Autodesk Fusion 360 part; units mm, degrees
(part 2 of 2)
sketch "Sketch5" plane through (-68.5, 0, 0) normal (-1, 0, 0) x (0, -1, 0) in component "Side"
  line L0 (-67.55, 105) -> (-67.55, 160)
  line L1 (-67.55, 160) -> (-77.55, 160)
  line L2 (-77.55, 160) -> (-77.55, 10)
  line L3 (-77.55, 10) -> (55.8, 10)
  line L4 (55.8, 10) -> (55.8, 20)
  line L5 (55.8, 20) -> (35.4, 20)
  arc A0 (20.4, 35) -> (35.4, 20) centre (35.4, 35) ccw
  line L6 (20.4, 35) -> (20.4, 88)
  arc A1 (20.4, 88) -> (18.4, 90) centre (18.4, 88) ccw
  line L7 (18.4, 90) -> (17.9998, 90)
  arc A2 (14.9998, 93) -> (17.9998, 90) centre (17.9998, 93) ccw
  line L8 (14.9998, 93) -> (14.9998, 112)
  arc A3 (14.9998, 112) -> (11.9998, 115) centre (11.9998, 112) ccw
  line L9 (11.9998, 115) -> (4.9998, 115)
  line L10 (4.9998, 115) -> (4.9998, 100)
  arc A4 (-5.0002, 100) -> (4.9998, 100) centre (-0.0002, 100) ccw
  line L11 (-5.0002, 100) -> (-5.0002, 115)
  line L12 (-5.0002, 115) -> (-12.0002, 115)
  arc A5 (-12.0002, 115) -> (-15.0002, 112) centre (-12.0002, 112) ccw
  line L13 (-15.0002, 112) -> (-15.0002, 95)
  arc A6 (-20.0002, 90) -> (-15.0002, 95) centre (-20.0002, 95) ccw
  line L14 (-20.0002, 90) -> (-52.55, 90)
  arc A7 (-67.55, 105) -> (-52.55, 90) centre (-52.55, 105) ccw
  line L15 (-0.0002, 95) -> (-0.0002, 10) construction
  line L16 (-25.4002, 90) -> (-25.4002, 10) construction
  line L17 (-50.8002, 90) -> (-50.8002, 10) construction
  line L18 (20.4, 30.4257) -> (-77.55, 30.4257) construction
  line L19 (20.4, 55.8257) -> (-77.55, 55.8257) construction
  line L20 (20.4, 81.2257) -> (-77.55, 81.2257) construction
  line L21 (-0.0002, 81.2257) -> (-50.8002, 30.4257) construction
  line L22 (-50.8002, 81.2257) -> (-0.0002, 30.4257) construction
  line L23 (-50.8002, 55.8257) -> (-25.4002, 81.2257) construction
  line L24 (-25.4002, 30.4257) -> (-0.0002, 55.8257) construction
  line L25 (-50.8002, 55.8257) -> (-25.4002, 30.4257) construction
  line L26 (-25.4002, 81.2257) -> (-0.0002, 55.8257) construction
  line L27 (-50.8002, 68.5257) -> (-0.0002, 68.5257) construction
  line L28 (-38.1002, 81.2257) -> (-38.1002, 30.4257) construction
  line L29 (-12.7002, 30.4257) -> (-12.7002, 81.2257) construction
  line L30 (-50.8002, 43.1257) -> (-0.0002, 43.1257) construction
  circle A8 centre (-50.8002, 81.2257) radius 3.1375
  circle A9 centre (-25.4002, 81.2257) radius 3.1375
  circle A10 centre (-0.0002, 81.2257) radius 3.1375
  circle A11 centre (-50.8002, 68.5257) radius 3.1375
  circle A12 centre (-25.4002, 68.5257) radius 3.1375
  circle A13 centre (-0.0002, 68.5257) radius 3.1375
  circle A14 centre (-50.8002, 55.8257) radius 3.1375
  circle A15 centre (-25.4002, 55.8257) radius 3.1375
  circle A16 centre (-0.0002, 55.8257) radius 3.1375
  circle A17 centre (-50.8002, 43.1257) radius 3.1375
  circle A18 centre (-38.1002, 81.2257) radius 3.1375
  circle A19 centre (-12.7002, 81.2257) radius 3.1375
  circle A20 centre (-38.1002, 68.5257) radius 3.1375
  circle A21 centre (-12.7002, 68.5257) radius 3.1375
  circle A22 centre (-38.1002, 55.8257) radius 3.1375
  circle A23 centre (-12.7002, 55.8257) radius 3.1375
  circle A24 centre (-38.1002, 43.1257) radius 3.1375
  circle A25 centre (-25.4002, 43.1257) radius 3.1375
  circle A26 centre (-12.7002, 43.1257) radius 3.1375
  circle A27 centre (-0.0002, 43.1257) radius 3.1375
  circle A28 centre (-0.0002, 30.4257) radius 3.1375
  circle A29 centre (-12.7002, 30.4257) radius 3.1375
  circle A30 centre (-25.4002, 30.4257) radius 3.1375
  circle A31 centre (-38.1002, 30.4257) radius 3.1375
  circle A32 centre (-50.8002, 30.4257) radius 3.1375
  line L31 (-77.55, 160) -> (-46.5335, 160)
  line L32 (-46.5335, 160) -> (-46.5335, 35)
  line L33 (-46.5335, 35) -> (-77.55, 35)
  line L34 (-77.55, 35) -> (-77.55, 160)
  dimension "d151" = 25.4
  dimension "d152" = 25.4
  dimension "d155" = 25.4
  dimension "d156" = 25.4
  dimension "d157" = 6.275
  dimension "d159" = 6.275
  dimension "d161" = 6.275
  dimension "d162" = 6.275
  dimension "d164" = 6.275
  dimension "d166" = 6.275
  dimension "d167" = 6.275
  dimension "d169" = 6.275
  dimension "d171" = 6.275
  dimension "d172" = 6.275
  dimension "d173" = 12.7
  dimension "d174" = 12.7
  dimension "d175" = 12.7
  dimension "d176" = 12.7
  dimension "d177" = 6.275
  dimension "d178" = 6.275
  dimension "d179" = 6.275
  dimension "d180" = 6.275
  dimension "d181" = 6.275
  dimension "d182" = 6.275
  dimension "d183" = 6.275
  dimension "d184" = 6.275
  dimension "d185" = 6.275
  dimension "d186" = 6.275
  dimension "d187" = 6.275
  dimension "d188" = 6.275
  dimension "d189" = 6.275
  dimension "d190" = 6.275
  dimension "d191" = 6.275
  dimension "d361" = 125
  constraint midpoint A4 L15.start
  constraint coincident L3 L15.end
  constraint perpendicular L3 L15
  constraint coincident L14 L16.start
  constraint coincident L3 L16.end
  constraint perpendicular L3 L16
  constraint coincident L14 L17.start
  constraint coincident L3 L17.end
  constraint perpendicular L3 L17
  constraint coincident L6 L18.start
  constraint coincident L2 L18.end
  constraint perpendicular L2 L18
  constraint coincident L6 L19.start
  constraint coincident L2 L19.end
  constraint perpendicular L2 L19
  constraint coincident L6 L20.start
  constraint coincident L2 L20.end
  constraint perpendicular L2 L20
  constraint coincident L15 L21.start
  constraint coincident L20 L21.start
  constraint coincident L18 L21.end
  constraint coincident L17 L21.end
  constraint coincident L17 L22.start
  constraint coincident L20 L22.start
  constraint coincident L18 L22.end
  constraint coincident L15 L22.end
  constraint coincident L19 L23.start
  constraint coincident L17 L23.start
  constraint coincident L20 L23.end
  constraint coincident L16 L23.end
  constraint coincident L18 L24.start
  constraint coincident L16 L24.start
  constraint coincident L19 L24.end
  constraint coincident L15 L24.end
  constraint coincident L17 L27.start
  constraint coincident L15 L27.end
  constraint perpendicular L15 L27
  constraint coincident L20 L28.start
  constraint coincident L18 L28.end
  constraint perpendicular L18 L28
  constraint coincident L18 L29.start
  constraint coincident L20 L29.end
  constraint perpendicular L20 L29
  constraint coincident L17 L30.start
  constraint coincident L15 L30.end
  constraint perpendicular L15 L30
  constraint coincident L22.start A8.centre
  constraint coincident L23.end L26.start
  constraint coincident L21.start A10.centre
  constraint coincident L27.start A11.centre
  constraint midpoint L27 A12.centre
  constraint coincident L27.end A13.centre
  constraint coincident L23.start L25.start
  constraint midpoint L21 A15.centre
  constraint coincident L24.end L26.end
  constraint coincident L30.start A17.centre
  constraint coincident L28.start A18.centre
  constraint coincident L29.end A19.centre
  constraint midpoint L23 A20.centre
  constraint midpoint L26 A21.centre
  constraint midpoint L28 A22.centre
  constraint midpoint L29 A23.centre
  constraint midpoint L25 A24.centre
  constraint midpoint L30 A25.centre
  constraint coincident L30 A26.centre
  constraint coincident L29 A26.centre
  constraint coincident L30.end A27.centre
  constraint coincident L22.end A28.centre
  constraint coincident L29.start A29.centre
  constraint coincident L24.start L25.end
  constraint coincident L28.end A31.centre
  constraint coincident L21.end A32.centre
  constraint horizontal L31
  constraint vertical L32
  constraint horizontal L33
  constraint vertical L34
  constraint coincident L1.end L2.start
  measures "d151" distance of L15 L16
  measures "d152" distance of L16 L17
  measures "d155" distance of L19 L20
  measures "d156" distance of L18 L19
  measures "d157" diameter of A8
  measures "d159" diameter of A9
  measures "d161" diameter of A10
  measures "d162" diameter of A11
  measures "d164" diameter of A12
  measures "d166" diameter of A13
  measures "d167" diameter of A14
  measures "d169" diameter of A15
  measures "d171" diameter of A16
  measures "d172" diameter of A17
  measures "d173" distance of L17 L28
  measures "d174" distance of L16 L29
  measures "d175" distance of L20 L27
  measures "d176" distance of L19 L30
  measures "d177" diameter of A18
  measures "d178" diameter of A19
  measures "d179" diameter of A20
  measures "d180" diameter of A21
  measures "d181" diameter of A22
  measures "d182" diameter of A23
  measures "d183" diameter of A24
  measures "d184" diameter of A25
  measures "d185" diameter of A26
  measures "d186" diameter of A27
  measures "d187" diameter of A28
  measures "d188" diameter of A29
  measures "d189" diameter of A30
  measures "d190" diameter of A31
  measures "d191" diameter of A32
  measures "d361" distance of L1.end L33.end
extrude "Extrude5" cut sketch "Sketch5" against normal up to surface (10 mm away) contours A8 | A9 | A10 | A11 | A12 | A13 | A14 | A15 | A16 | A17 | A18 | A19 | A20 | A21 | A22 | A23 | A24 | A25 | A26 | A27 | A28 | A29 | A30 | A31 | A32 bodies 3 in component "Side"
sketch "Sketch6" plane through (0, -14.9998, 0) normal (0, -1, 0) x (1, 0, 0) in component "Side"
  line L0 (-58.5, 93) -> (-58.5, 112)
  line L1 (-58.5, 112) -> (-68.5, 112)
  line L2 (-68.5, 112) -> (-68.5, 93)
  line L3 (-68.5, 93) -> (-58.5, 93)
  line L4 (-58.5, 112) -> (-68.5, 93) construction
  line L5 (-68.5, 112) -> (-58.5, 93) construction
  circle A0 centre (-63.5, 102.5) radius 3.1375
  dimension "d194" = 6.275
  constraint coincident L0.end L1.start
  constraint coincident L2.end L3.start
  constraint coincident L1.end L2.start
  constraint coincident L0.start L3.end
  constraint midpoint L5 A0.centre
  measures "d194" diameter of A0
extrude "Extrude6" cut sketch "Sketch6" against normal up to surface (3 mm away) contours A0 bodies 3 in component "Side"
sketch "Sketch7" plane through (0, 77.55, 0) normal (0, 1, 0) x (-1, 0, 0) in component "Side"
  line L0 (58.5, 10) -> (68.5, 10)
  line L1 (68.5, 10) -> (68.5, 160)
  line L2 (68.5, 160) -> (58.5, 160)
  line L3 (58.5, 160) -> (58.5, 10)
  line L4 (68.5, 160) -> (58.5, 10) construction
  line L5 (58.5, 160) -> (68.5, 10) construction
  line L6 (58.5, 85) -> (68.5, 85) construction
  line L7 (58.5, 85) -> (68.5, 160) construction
  line L8 (58.5, 160) -> (68.5, 85) construction
  line L9 (68.5, 85) -> (58.5, 10) construction
  line L10 (58.5, 85) -> (68.5, 10) construction
  circle A0 centre (63.5, 47.5) radius 3.1375
  circle A1 centre (63.5, 85) radius 3.1375
  circle A2 centre (63.5, 122.5) radius 3.1375
  dimension "d197" = 6.275
  dimension "d198" = 6.275
  dimension "d199" = 6.275
  constraint coincident L1.end L2.start
  constraint coincident L0.start L3.end
  constraint coincident L2.end L3.start
  constraint coincident L0.end L1.start
  constraint midpoint L3 L6.start
  constraint midpoint L1 L6.end
  constraint midpoint L9 A0.centre
  constraint midpoint L4 A1.centre
  constraint midpoint L8 A2.centre
  measures "d197" diameter of A0
  measures "d198" diameter of A1
  measures "d199" diameter of A2
extrude "Extrude7" cut sketch "Sketch7" against normal blind 22.5 contours A0 | A1 | A2 bodies 3 in component "Side"
sketch "Sketch3 (2)" plane through (0, 77.55, 0) normal (0, -1, 0) x (1, 0, 0) in component "Back"
  line L0 (-68.5, 10) -> (68.5, 10)
  line L1 (68.5, 10) -> (68.5, 160)
  line L2 (68.5, 160) -> (-68.5, 160)
  line L3 (-68.5, 160) -> (-68.5, 10)
  line L4 (-58.5, 160) -> (-58.5, 10) construction
  line L5 (58.5, 160) -> (58.5, 10) construction
  line L6 (-58.5, 160) -> (-68.5, 10) construction
  line L7 (-68.5, 160) -> (-58.5, 10) construction
  line L8 (-68.5, 85) -> (-58.5, 160) construction
  line L9 (-68.5, 160) -> (-58.5, 85) construction
  line L10 (-58.5, 85) -> (-68.5, 10) construction
  line L11 (-68.5, 85) -> (-58.5, 10) construction
  circle A0 centre (-63.5, 47.5) radius 3.35
  line L12 (68.5, 160) -> (58.5, 10) construction
  line L13 (58.5, 160) -> (68.5, 10) construction
  line L14 (58.5, 85) -> (68.5, 160) construction
  line L15 (58.5, 160) -> (68.5, 85) construction
  line L16 (68.5, 85) -> (58.5, 10) construction
  line L17 (58.5, 85) -> (68.5, 10) construction
  circle A1 centre (63.5, 47.5) radius 3.35
  line L18 (0, 160) -> (0, 10) construction
  line L19 (25.4, 160) -> (25.4, 10) construction
  line L20 (50.8, 160) -> (50.8, 10) construction
  line L21 (-25.4, 160) -> (-25.4, 10) construction
  line L22 (-50.8, 160) -> (-50.8, 10) construction
  line L23 (-68.5, 147.9) -> (68.5, 147.9) construction
  line L24 (-63.5, 122.5) -> (63.5, 122.5) construction
  line L25 (-68.5, 97.1) -> (68.5, 97.1) construction
  line L26 (-68.5, 46.3) -> (68.5, 46.3) construction
  line L27 (-68.5, 20.9) -> (68.5, 20.9) construction
  line L28 (-68.5, 71.7) -> (68.5, 71.7) construction
  line L29 (-50.8, 147.9) -> (50.8, 46.3) construction
  line L30 (-50.8, 122.5) -> (50.8, 20.9) construction
  line L31 (50.8, 147.9) -> (-50.8, 46.3) construction
  line L32 (50.8, 122.5) -> (-50.8, 20.9) construction
  line L33 (25.4, 147.9) -> (-50.8, 71.7) construction
  line L34 (0, 147.9) -> (-50.8, 97.1) construction
  line L35 (-25.4, 147.9) -> (-50.8, 122.5) construction
  line L36 (-25.4, 147.9) -> (50.8, 71.7) construction
  line L37 (0, 147.9) -> (50.8, 97.1) construction
  line L38 (25.4, 147.9) -> (50.8, 122.5) construction
  line L39 (-50.8, 97.1) -> (25.4, 20.9) construction
  line L40 (-50.8, 71.7) -> (0, 20.9) construction
  line L41 (-50.8, 46.3) -> (-25.4, 20.9) construction
  line L42 (-25.4, 20.9) -> (50.8, 97.1) construction
  line L43 (0, 20.9) -> (50.8, 71.7) construction
  line L44 (25.4, 20.9) -> (50.8, 46.3) construction
  circle A2 centre (-50.8, 46.3) radius 3.1375
  circle A3 centre (-25.4, 46.3) radius 3.1375
  circle A4 centre (0, 46.3) radius 3.1375
  circle A5 centre (25.4, 46.3) radius 3.1375
  circle A6 centre (50.8, 46.3) radius 3.1375
  circle A7 centre (-50.8, 20.9) radius 3.1375
  circle A8 centre (-25.4, 20.9) radius 3.1375
  circle A9 centre (0, 20.9) radius 3.1375
  circle A10 centre (25.4, 20.9) radius 3.1375
  circle A11 centre (50.8, 20.9) radius 3.1375
  circle A12 centre (-38.1, 33.6) radius 3.1375
  circle A13 centre (-12.7, 33.6) radius 3.1375
  circle A14 centre (12.7, 33.6) radius 3.1375
  circle A15 centre (38.1, 33.6) radius 3.1375
  circle A16 centre (63.5, 47.5) radius 5
  circle A17 centre (-63.5, 47.5) radius 5
  dimension "d202" = 10
  dimension "d203" = 10
  dimension "d206" = 6.7
  dimension "d209" = 6.7
  dimension "d210" = 25.4
  dimension "d211" = 25.4
  dimension "d212" = 25.4
  dimension "d213" = 25.4
  dimension "d214" = 25.4
  dimension "d215" = 25.4
  dimension "d216" = 25.4
  dimension "d217" = 25.4
  dimension "d218" = 25.4
  dimension "d239" = 6.275
  dimension "d240" = 6.275
  dimension "d241" = 6.275
  dimension "d242" = 6.275
  dimension "d243" = 6.275
  dimension "d244" = 6.275
  dimension "d245" = 6.275
  dimension "d246" = 6.275
  dimension "d247" = 6.275
  dimension "d248" = 6.275
  dimension "d265" = 6.275
  dimension "d266" = 6.275
  dimension "d267" = 6.275
  dimension "d268" = 6.275
  dimension "d351" = 10
  dimension "d354" = 10
  constraint coincident L2 L4.start
  constraint coincident L0 L4.end
  constraint perpendicular L0 L4
  constraint coincident L2 L5.start
  constraint coincident L0 L5.end
  constraint perpendicular L0 L5
  constraint coincident L0.start L3.end
  constraint coincident L2.end L3.start
  constraint midpoint L3 L8.start
  constraint midpoint L1 L15.end
  constraint midpoint L4 L9.end
  constraint midpoint L11 A0.centre
  constraint coincident L1.end L2.start
  constraint coincident L0.end L1.start
  constraint midpoint L5 L14.start
  constraint midpoint L17 A1.centre
  constraint midpoint L2 L18.start
  constraint midpoint L0 L18.end
  constraint coincident L2 L19.start
  constraint coincident L0 L19.end
  constraint perpendicular L0 L19
  constraint coincident L2 L20.start
  constraint coincident L0 L20.end
  constraint perpendicular L0 L20
  constraint coincident L2 L21.start
  constraint coincident L0 L21.end
  constraint perpendicular L0 L21
  constraint coincident L2 L22.start
  constraint coincident L0 L22.end
  constraint perpendicular L0 L22
  constraint coincident L3 L23.start
  constraint coincident L1 L23.end
  constraint perpendicular L1 L23
  constraint coincident L3 L25.start
  constraint coincident L1 L25.end
  constraint perpendicular L1 L25
  constraint coincident L3 L26.start
  constraint coincident L1 L26.end
  constraint perpendicular L1 L26
  constraint coincident L3 L27.start
  constraint coincident L1 L27.end
  constraint perpendicular L1 L27
  constraint coincident L3 L28.start
  constraint coincident L1 L28.end
  constraint perpendicular L1 L28
  constraint coincident L23 L29.start
  constraint coincident L22 L29.start
  constraint coincident L26 L29.end
  constraint coincident L20 L29.end
  constraint coincident L22 L30.start
  constraint coincident L24 L30.start
  constraint coincident L27 L30.end
  constraint coincident L20 L30.end
  constraint coincident L23 L31.start
  constraint coincident L20 L31.start
  constraint coincident L26 L31.end
  constraint coincident L22 L31.end
  constraint coincident L20 L32.start
  constraint coincident L24 L32.start
  constraint coincident L22 L32.end
  constraint coincident L27 L32.end
  constraint coincident L19 L33.start
  constraint coincident L23 L33.start
  constraint coincident L28 L33.end
  constraint coincident L22 L33.end
  constraint midpoint L23 L34.start
  constraint coincident L25 L34.end
  constraint coincident L22 L34.end
  constraint coincident L23 L35.start
  constraint coincident L21 L35.start
  constraint coincident L28 L36.end
  constraint coincident L20 L36.end
  constraint coincident L25 L37.end
  constraint coincident L20 L37.end
  constraint coincident L27 L39.end
  constraint coincident L19 L39.end
  constraint midpoint L27 L40.end
  constraint coincident L21 L41.end
  constraint coincident L27 L41.end
  constraint coincident L31.end L41.start
  constraint midpoint L40 A3.centre
  constraint midpoint L26 A4.centre
  constraint midpoint L43 A5.centre
  constraint coincident L29.end L44.end
  constraint coincident L32.end A7.centre
  constraint coincident L41.end L42.start
  constraint coincident L40.end L43.start
  constraint coincident L39.end L44.start
  constraint coincident L30.end A11.centre
  constraint midpoint L41 A12.centre
  constraint coincident L42 A13.centre
  constraint coincident L40 A13.centre
  constraint coincident L43 A14.centre
  constraint coincident L39 A14.centre
  constraint midpoint L44 A15.centre
  constraint concentric A1 A16
  constraint concentric A0 A17
  measures "d202" distance of L3 L4
  measures "d203" distance of L1 L5
  measures "d206" diameter of A0
  measures "d209" diameter of A1
  measures "d210" distance of L18 L19
  measures "d211" distance of L19 L20
  measures "d212" distance of L18 L21
  measures "d213" distance of L21 L22
  measures "d214" distance of L23 L24
  measures "d215" distance of L24 L25
  measures "d216" distance of L25 L28
  measures "d217" distance of L26 L28
  measures "d218" distance of L26 L27
  measures "d239" diameter of A2
  measures "d240" diameter of A3
  measures "d241" diameter of A4
  measures "d242" diameter of A5
  measures "d243" diameter of A6
  measures "d244" diameter of A7
  measures "d245" diameter of A8
  measures "d246" diameter of A9
  measures "d247" diameter of A10
  measures "d248" diameter of A11
  measures "d265" diameter of A12
  measures "d266" diameter of A13
  measures "d267" diameter of A14
  measures "d268" diameter of A15
  measures "d351" diameter of A16
  measures "d354" diameter of A17
extrude "Extrude3'" cut sketch "Sketch3 (2)" against normal up to surface (10 mm away) contours A0 | A1 | A2 | A3 | A4 | A5 | A6 | A7 | A8 | A9 | A10 | A11 | A12 | A13 | A14 | A15 bodies 2 in component "Back"
sketch "Sketch1 (4)" plane through (0, 0, 10) normal (0, 0, 1) x (-1, 0, 0) in component "Plate"
  circle A0 centre (-12.7, 25.4) radius 3.1375
  circle A1 centre (12.7, 25.4) radius 3.1375
  line L0 (76.55, -65) -> (75.85, -65)
  arc A2 (72.85, -62) -> (75.85, -65) centre (75.85, -62) ccw
  line L1 (72.85, -62) -> (72.85, 62)
  arc A3 (75.85, 65) -> (72.85, 62) centre (75.85, 62) ccw
  line L2 (75.85, 65) -> (76.55, 65)
  arc A4 (79.55, 62) -> (76.55, 65) centre (76.55, 62) ccw
  line L3 (79.55, 62) -> (79.55, -62)
  arc A5 (76.55, -65) -> (79.55, -62) centre (76.55, -62) ccw
  arc A6 (-76.55, 65) -> (-79.55, 62) centre (-76.55, 62) ccw
  line L4 (-76.55, 65) -> (-75.85, 65)
  arc A7 (-72.85, 62) -> (-75.85, 65) centre (-75.85, 62) ccw
  line L5 (-72.85, 62) -> (-72.85, -62)
  arc A8 (-75.85, -65) -> (-72.85, -62) centre (-75.85, -62) ccw
  line L6 (-75.85, -65) -> (-76.55, -65)
  arc A9 (-79.55, -62) -> (-76.55, -65) centre (-76.55, -62) ccw
  line L7 (-79.55, -62) -> (-79.55, 62)
  circle A10 centre (-63.5, 50.8) radius 3.1375
  circle A11 centre (-38.1, 50.8) radius 3.1375
  circle A12 centre (-12.7, 50.8) radius 3.1375
  circle A13 centre (12.7, 50.8) radius 3.1375
  circle A14 centre (38.1, 50.8) radius 3.1375
  circle A15 centre (63.5, 50.8) radius 3.1375
  circle A16 centre (-63.5, 25.4) radius 3.1375
  circle A17 centre (-38.1, 25.4) radius 3.1375
  circle A18 centre (12.7, -50.8) radius 3.1375
  circle A19 centre (-12.7, -50.8) radius 3.1375
  circle A20 centre (-38.1, -50.8) radius 3.1375
  circle A21 centre (-63.5, -50.8) radius 3.1375
  circle A22 centre (63.5, -25.4) radius 3.1375
  circle A23 centre (38.1, -25.4) radius 3.1375
  circle A24 centre (12.7, -25.4) radius 3.1375
  circle A25 centre (-63.5, 0) radius 3.1375
  circle A26 centre (63.5, 25.4) radius 3.1375
  circle A27 centre (38.1, 25.4) radius 3.1375
  circle A28 centre (38.1, -50.8) radius 3.1375
  circle A29 centre (63.5, -50.8) radius 3.1375
  circle A30 centre (-63.5, 82.55) radius 3.1375
  circle A31 centre (-38.1, 82.55) radius 3.1375
  circle A32 centre (-12.7, 82.55) radius 3.1375
  circle A33 centre (12.7, 82.55) radius 3.1375
  circle A34 centre (38.1, 82.55) radius 3.1375
  circle A35 centre (63.5, 82.55) radius 3.1375
  circle A36 centre (-63.5, -82.55) radius 3.1375
  circle A37 centre (-38.1, -82.55) radius 3.1375
  circle A38 centre (-12.7, -82.55) radius 3.1375
  circle A39 centre (12.7, -82.55) radius 3.1375
  circle A40 centre (38.1, -82.55) radius 3.1375
  circle A41 centre (63.5, -82.55) radius 3.1375
  circle A42 centre (-63.5, -25.4) radius 3.1375
  circle A43 centre (-12.7, -25.4) radius 3.1375
  circle A44 centre (-38.1, 0) radius 3.1375
  circle A45 centre (38.1, 0) radius 3.1375
  circle A46 centre (-12.7, 0) radius 3.1375
  circle A47 centre (-38.1, -25.4) radius 3.1375
  circle A48 centre (63.5, 0) radius 3.1375
  circle A49 centre (12.7, 0) radius 3.1375
  line L8 (-79.2, 76.2) -> (-85.9, 76.2)
  arc A50 (-85.9, 76.2) -> (-88.9, 73.2) centre (-85.9, 73.2) ccw
  line L9 (-88.9, 73.2) -> (-88.9, -73.2)
  arc A51 (-88.9, -73.2) -> (-85.9, -76.2) centre (-85.9, -73.2) ccw
  line L10 (-85.9, -76.2) -> (-79.2, -76.2)
  arc A52 (-76.2, -79.2) -> (-79.2, -76.2) centre (-79.2, -79.2) ccw
  line L11 (-76.2, -79.2) -> (-76.2, -85.9)
  arc A53 (-76.2, -85.9) -> (-73.2, -88.9) centre (-73.2, -85.9) ccw
  line L12 (-73.2, -88.9) -> (73.2, -88.9)
  arc A54 (73.2, -88.9) -> (76.2, -85.9) centre (73.2, -85.9) ccw
  line L13 (76.2, -85.9) -> (76.2, -79.2)
  arc A55 (79.2, -76.2) -> (76.2, -79.2) centre (79.2, -79.2) ccw
  line L14 (79.2, -76.2) -> (85.9, -76.2)
  arc A56 (85.9, -76.2) -> (88.9, -73.2) centre (85.9, -73.2) ccw
  line L15 (88.9, -73.2) -> (88.9, 73.2)
  arc A57 (88.9, 73.2) -> (85.9, 76.2) centre (85.9, 73.2) ccw
  line L16 (85.9, 76.2) -> (79.2, 76.2)
  arc A58 (76.2, 79.2) -> (79.2, 76.2) centre (79.2, 79.2) ccw
  line L17 (76.2, 79.2) -> (76.2, 85.9)
  arc A59 (76.2, 85.9) -> (73.2, 88.9) centre (73.2, 85.9) ccw
  line L18 (73.2, 88.9) -> (-73.2, 88.9)
  arc A60 (-73.2, 88.9) -> (-76.2, 85.9) centre (-73.2, 85.9) ccw
  line L19 (-76.2, 85.9) -> (-76.2, 79.2)
  arc A61 (-79.2, 76.2) -> (-76.2, 79.2) centre (-79.2, 79.2) ccw
  line L20 (0, 0) -> (-73.2, 85.9) construction
  line L21 (0, 0) -> (-73.2, -85.9) construction
  line L22 (0, 0) -> (73.2, -85.9) construction
  line L23 (0, 0) -> (73.2, 85.9) construction
  line L24 (57.5, 76.75) -> (-57.5, 76.75)
  line L25 (-57.5, 76.75) -> (-57.5, -76.75)
  line L26 (-57.5, -76.75) -> (57.5, -76.75)
  line L27 (57.5, -76.75) -> (57.5, 76.75)
  line L28 (57.5, 76.75) -> (-57.5, -76.75) construction
  line L29 (-57.5, 76.75) -> (57.5, -76.75) construction
  line L30 (38.1, -50.8) -> (-38.1, -50.8) construction
  line L31 (-38.1, -50.8) -> (-38.1, 50.8) construction
  line L32 (-38.1, 50.8) -> (38.1, 50.8) construction
  line L33 (38.1, 50.8) -> (38.1, -50.8) construction
  line L34 (38.1, -25.4) -> (-38.1, -25.4) construction
  line L35 (38.1, 0) -> (-38.1, 0) construction
  line L36 (38.1, 25.4) -> (-38.1, 25.4) construction
  line L37 (12.7, 50.8) -> (12.7, -50.8) construction
  line L38 (-12.7, -50.8) -> (-12.7, 50.8) construction
  circle A62 centre (38.1, 50.8) radius 3.05
  circle A63 centre (12.7, 50.8) radius 3.05
  circle A64 centre (-12.7, 50.8) radius 3.05
  circle A65 centre (-38.1, 50.8) radius 3.05
  circle A66 centre (38.1, 25.4) radius 3.05
  circle A67 centre (12.7, 25.4) radius 3.05
  circle A68 centre (-12.7, 25.4) radius 3.05
  circle A69 centre (-38.1, 25.4) radius 3.05
  circle A70 centre (38.1, 0) radius 3.05
  circle A71 centre (12.7, 0) radius 3.05
  circle A72 centre (-12.7, 0) radius 3.05
  circle A73 centre (-38.1, 0) radius 3.05
  circle A74 centre (38.1, -25.4) radius 3.05
  circle A75 centre (12.7, -25.4) radius 3.05
  circle A76 centre (-12.7, -25.4) radius 3.05
  circle A77 centre (-38.1, -25.4) radius 3.05
  circle A78 centre (38.1, -50.8) radius 3.05
  circle A79 centre (12.7, -50.8) radius 3.05
  circle A80 centre (-12.7, -50.8) radius 3.05
  circle A81 centre (-38.1, -50.8) radius 3.05
  dimension "d271" = 153.5
  dimension "d272" = 115
  dimension "d275" = 6.1
  dimension "d276" = 6.1
  dimension "d277" = 6.1
  dimension "d278" = 6.1
  dimension "d279" = 6.1
  dimension "d280" = 6.1
  dimension "d281" = 6.1
  dimension "d282" = 6.1
  dimension "d283" = 6.1
  dimension "d284" = 6.1
  dimension "d285" = 6.1
  dimension "d286" = 6.1
  dimension "d287" = 6.1
  dimension "d288" = 6.1
  dimension "d289" = 6.1
  dimension "d290" = 6.1
  dimension "d291" = 6.1
  dimension "d292" = 6.1
  dimension "d293" = 6.1
  dimension "d294" = 6.1
  constraint coincident L20.start L21.start
  constraint coincident A60.centre L20.end
  constraint coincident A53.centre L21.end
  constraint coincident A54.centre L22.end
  constraint coincident A59.centre L23.end
  constraint perpendicular L24 L25
  constraint parallel L24 L26
  constraint parallel L25 L27
  constraint horizontal L24
  constraint coincident L28 L20.start
  constraint coincident L29 L20.start
  constraint coincident A28.centre L30.start
  constraint coincident A20.centre L30.end
  constraint coincident A11.centre L31.end
  constraint coincident A14.centre L32.end
  constraint coincident A23.centre L34.start
  constraint coincident A47.centre L34.end
  constraint coincident A45.centre L35.start
  constraint coincident A44.centre L35.end
  constraint coincident A27.centre L36.start
  constraint coincident A17.centre L36.end
  constraint coincident A13.centre L37.start
  constraint coincident A18.centre L37.end
  constraint coincident A19.centre L38.start
  constraint coincident A12.centre L38.end
  constraint concentric A13 A63
  constraint concentric A11 A65
  constraint concentric A1 A67
  constraint concentric A0 A68
  constraint concentric A17 A69
  constraint concentric A49 A71
  constraint concentric A46 A72
  constraint concentric A44 A73
  constraint concentric A24 A75
  constraint concentric A43 A76
  constraint concentric A28 A78
  constraint concentric A19 A80
  measures "d271" distance of L24.end L25.end
  measures "d272" distance of L25.end L26.end
  measures "d275" diameter of A62
  measures "d276" diameter of A63
  measures "d277" diameter of A64
  measures "d278" diameter of A65
  measures "d279" diameter of A66
  measures "d280" diameter of A67
  measures "d281" diameter of A68
  measures "d282" diameter of A69
  measures "d283" diameter of A70
  measures "d284" diameter of A71
  measures "d285" diameter of A72
  measures "d286" diameter of A73
  measures "d287" diameter of A74
  measures "d288" diameter of A75
  measures "d289" diameter of A76
  measures "d290" diameter of A77
  measures "d291" diameter of A78
  measures "d292" diameter of A79
  measures "d293" diameter of A80
  measures "d294" diameter of A81
extrude "Extrude1'''" add sketch "Sketch1 (4)" along normal blind 3.2 separate body contours A0 | A1 | A11 | A12 | A13 | A14 | A17 | A18 | A19 | A20 | A23 | A24 | A27 | A28 | A43 | A44 | A45 | A46 | A47 | A49 | L24 L25 L26 L27 | A62 | A63 | A64 | A65 | A66 | A67 | A68 | A69 | A70 | A71 | A72 | A73 | A74 | A75 | A76 | A77 | A78 | A79 | A80 | A81 makes body 4 in component "Plate"
extrude "Extrude2''" add sketch "Sketch1 (4)" against normal blind 3 contours A62 | A63 | A64 | A65 | A66 | A67 | A68 | A69 | A70 | A71 | A72 | A73 | A74 | A75 | A76 | A77 | A78 | A79 | A80 | A81 bodies 4 in component "Plate"
sketch "Sketch2 (3)" plane through (0, 0, 13.2) normal (0, 0, 1) x (-1, 0, 0) in component "Plate"
  line L0 (57.5, -76.75) -> (57.5, 76.75)
  line L1 (57.5, 76.75) -> (-57.5, 76.75)
  line L2 (-57.5, 76.75) -> (-57.5, -76.75)
  line L3 (-57.5, -76.75) -> (57.5, -76.75)
  line L4 (-55, 74.25) -> (55, 74.25)
  line L5 (55, 74.25) -> (55, -74.25)
  line L6 (55, -74.25) -> (-55, -74.25)
  line L7 (-55, -74.25) -> (-55, 74.25)
  line L8 (-55, 74.25) -> (55, -74.25) construction
  line L9 (55, 74.25) -> (-55, -74.25) construction
  dimension "d297" = 110
  dimension "d298" = 148.5
  constraint perpendicular L4 L5
  constraint parallel L4 L6
  constraint parallel L5 L7
  constraint horizontal L4
  constraint coincident L8 origin
  constraint coincident L9 origin
  measures "d297" distance of L5.end L6.end
  measures "d298" distance of L4.end L5.end
extrude "Extrude3''" cut sketch "Sketch2 (3)" against normal blind 1.5 contours L4 L5 L6 L7 bodies 4 in component "Plate"
sketch "Sketch2 (4)" plane through (0, 0, 0) normal (0, 0, -1) x (1, 0, 0)
  circle A0 centre (12.7, 25.4) radius 3.1375
  circle A1 centre (-12.7, 25.4) radius 3.1375
  line L0 (-75.85, -65) -> (-76.55, -65)
  arc A2 (-79.55, -62) -> (-76.55, -65) centre (-76.55, -62) ccw
  line L1 (-79.55, -62) -> (-79.55, 62)
  arc A3 (-76.55, 65) -> (-79.55, 62) centre (-76.55, 62) ccw
  line L2 (-76.55, 65) -> (-75.85, 65)
  arc A4 (-72.85, 62) -> (-75.85, 65) centre (-75.85, 62) ccw
  line L3 (-72.85, 62) -> (-72.85, -62)
  arc A5 (-75.85, -65) -> (-72.85, -62) centre (-75.85, -62) ccw
  arc A6 (79.55, 62) -> (76.55, 65) centre (76.55, 62) ccw
  line L4 (79.55, 62) -> (79.55, -62)
  arc A7 (76.55, -65) -> (79.55, -62) centre (76.55, -62) ccw
  line L5 (76.55, -65) -> (75.85, -65)
  arc A8 (72.85, -62) -> (75.85, -65) centre (75.85, -62) ccw
  line L6 (72.85, -62) -> (72.85, 62)
  arc A9 (75.85, 65) -> (72.85, 62) centre (75.85, 62) ccw
  line L7 (75.85, 65) -> (76.55, 65)
  circle A10 centre (63.5, 50.8) radius 3.1375
  circle A11 centre (38.1, 50.8) radius 3.1375
  circle A12 centre (12.7, 50.8) radius 3.1375
  circle A13 centre (-12.7, 50.8) radius 3.1375
  circle A14 centre (-38.1, 50.8) radius 3.1375
  circle A15 centre (-63.5, 50.8) radius 3.1375
  circle A16 centre (63.5, 25.4) radius 3.1375
  circle A17 centre (38.1, 25.4) radius 3.1375
  circle A18 centre (-12.7, -50.8) radius 3.1375
  circle A19 centre (12.7, -50.8) radius 3.1375
  circle A20 centre (38.1, -50.8) radius 3.1375
  circle A21 centre (63.5, -50.8) radius 3.1375
  circle A22 centre (-63.5, -25.4) radius 3.1375
  circle A23 centre (-38.1, -25.4) radius 3.1375
  circle A24 centre (-12.7, -25.4) radius 3.1375
  circle A25 centre (63.5, 0) radius 3.1375
  circle A26 centre (-63.5, 25.4) radius 3.1375
  circle A27 centre (-38.1, 25.4) radius 3.1375
  circle A28 centre (-38.1, -50.8) radius 3.1375
  circle A29 centre (-63.5, -50.8) radius 3.1375
  circle A30 centre (63.5, 82.55) radius 3.1375
  circle A31 centre (38.1, 82.55) radius 3.1375
  circle A32 centre (12.7, 82.55) radius 3.1375
  circle A33 centre (-12.7, 82.55) radius 3.1375
  circle A34 centre (-38.1, 82.55) radius 3.1375
  circle A35 centre (-63.5, 82.55) radius 3.1375
  circle A36 centre (63.5, -82.55) radius 3.1375
  circle A37 centre (38.1, -82.55) radius 3.1375
  circle A38 centre (12.7, -82.55) radius 3.1375
  circle A39 centre (-12.7, -82.55) radius 3.1375
  circle A40 centre (-38.1, -82.55) radius 3.1375
  circle A41 centre (-63.5, -82.55) radius 3.1375
  circle A42 centre (63.5, -25.4) radius 3.1375
  circle A43 centre (12.7, -25.4) radius 3.1375
  circle A44 centre (38.1, 0) radius 3.1375
  circle A45 centre (-38.1, 0) radius 3.1375
  circle A46 centre (12.7, 0) radius 3.1375
  circle A47 centre (38.1, -25.4) radius 3.1375
  circle A48 centre (-63.5, 0) radius 3.1375
  circle A49 centre (-12.7, 0) radius 3.1375
  line L8 (85.9, 76.2) -> (79.2, 76.2)
  arc A50 (76.2, 79.2) -> (79.2, 76.2) centre (79.2, 79.2) ccw
  line L9 (76.2, 79.2) -> (76.2, 85.9)
  arc A51 (76.2, 85.9) -> (73.2, 88.9) centre (73.2, 85.9) ccw
  line L10 (73.2, 88.9) -> (-73.2, 88.9)
  arc A52 (-73.2, 88.9) -> (-76.2, 85.9) centre (-73.2, 85.9) ccw
  line L11 (-76.2, 85.9) -> (-76.2, 79.2)
  arc A53 (-79.2, 76.2) -> (-76.2, 79.2) centre (-79.2, 79.2) ccw
  line L12 (-79.2, 76.2) -> (-85.9, 76.2)
  arc A54 (-85.9, 76.2) -> (-88.9, 73.2) centre (-85.9, 73.2) ccw
  line L13 (-88.9, 73.2) -> (-88.9, -73.2)
  arc A55 (-88.9, -73.2) -> (-85.9, -76.2) centre (-85.9, -73.2) ccw
  line L14 (-85.9, -76.2) -> (-79.2, -76.2)
  arc A56 (-76.2, -79.2) -> (-79.2, -76.2) centre (-79.2, -79.2) ccw
  line L15 (-76.2, -79.2) -> (-76.2, -85.9)
  arc A57 (-76.2, -85.9) -> (-73.2, -88.9) centre (-73.2, -85.9) ccw
  line L16 (-73.2, -88.9) -> (73.2, -88.9)
  arc A58 (73.2, -88.9) -> (76.2, -85.9) centre (73.2, -85.9) ccw
  line L17 (76.2, -85.9) -> (76.2, -79.2)
  arc A59 (79.2, -76.2) -> (76.2, -79.2) centre (79.2, -79.2) ccw
  line L18 (79.2, -76.2) -> (85.9, -76.2)
  arc A60 (85.9, -76.2) -> (88.9, -73.2) centre (85.9, -73.2) ccw
  line L19 (88.9, -73.2) -> (88.9, 73.2)
  arc A61 (88.9, 73.2) -> (85.9, 76.2) centre (85.9, 73.2) ccw
  circle A62 centre (-63.5, -82.55) radius 3.35
  circle A63 centre (-38.1, -82.55) radius 3.35
  circle A64 centre (-12.7, -82.55) radius 3.35
  circle A65 centre (12.7, -82.55) radius 3.35
  circle A66 centre (38.1, -82.55) radius 3.35
  circle A67 centre (63.5, -82.55) radius 3.35
  circle A68 centre (63.5, -50.8) radius 3.35
  circle A69 centre (63.5, -25.4) radius 3.35
  circle A70 centre (63.5, 0) radius 3.35
  circle A71 centre (63.5, 25.4) radius 3.35
  circle A72 centre (63.5, 50.8) radius 3.35
  circle A73 centre (-63.5, -50.8) radius 3.35
  circle A74 centre (-63.5, -25.4) radius 3.35
  circle A75 centre (-63.5, 0) radius 3.35
  circle A76 centre (-63.5, 25.4) radius 3.35
  circle A77 centre (-63.5, 50.8) radius 3.35
  circle A78 centre (-63.5, 82.55) radius 3.35
  circle A79 centre (-38.1, 82.55) radius 3.35
  circle A80 centre (-12.7, 82.55) radius 3.35
  circle A81 centre (12.7, 82.55) radius 3.35
  circle A82 centre (38.1, 82.55) radius 3.35
  circle A83 centre (63.5, 82.55) radius 3.35
  circle A84 centre (-63.5, 82.55) radius 5
  circle A85 centre (-38.1, 82.55) radius 5
  circle A86 centre (-12.7, 82.55) radius 5
  circle A87 centre (12.7, 82.55) radius 5
  circle A88 centre (38.1, 82.55) radius 5
  circle A89 centre (63.5, 82.55) radius 5
  circle A90 centre (63.5, 50.8) radius 5
  circle A91 centre (63.5, 25.4) radius 5
  circle A92 centre (63.5, 0) radius 5
  circle A93 centre (63.5, -25.4) radius 5
  circle A94 centre (63.5, -50.8) radius 5
  circle A95 centre (63.5, -82.55) radius 5
  circle A96 centre (38.1, -82.55) radius 5
  circle A97 centre (12.7, -82.55) radius 5
  circle A98 centre (-12.7, -82.55) radius 5
  circle A99 centre (-38.1, -82.55) radius 5
  circle A100 centre (-63.5, -82.55) radius 5
  circle A101 centre (-63.5, -50.8) radius 5
  circle A102 centre (-63.5, -25.4) radius 5
  circle A103 centre (-63.5, 0) radius 5
  circle A104 centre (-63.5, 25.4) radius 5
  circle A105 centre (-63.5, 50.8) radius 5
  dimension "d301" = 6.7
  dimension "d302" = 6.7
  dimension "d303" = 6.7
  dimension "d304" = 6.7
  dimension "d305" = 6.7
  dimension "d306" = 6.7
  dimension "d307" = 6.7
  dimension "d308" = 6.7
  dimension "d309" = 6.7
  dimension "d310" = 6.7
  dimension "d311" = 6.7
  dimension "d312" = 6.7
  dimension "d313" = 6.7
  dimension "d314" = 6.7
  dimension "d315" = 6.7
  dimension "d316" = 6.7
  dimension "d317" = 6.7
  dimension "d318" = 6.7
  dimension "d319" = 6.7
  dimension "d320" = 6.7
  dimension "d321" = 6.7
  dimension "d322" = 6.7
  dimension "d325" = 10
  dimension "d326" = 10
  dimension "d327" = 10
  dimension "d328" = 10
  dimension "d329" = 10
  dimension "d330" = 10
  dimension "d331" = 10
  dimension "d332" = 10
  dimension "d333" = 10
  dimension "d334" = 10
  dimension "d335" = 10
  dimension "d336" = 10
  dimension "d337" = 10
  dimension "d338" = 10
  dimension "d339" = 10
  dimension "d340" = 10
  dimension "d341" = 10
  dimension "d342" = 10
  dimension "d343" = 10
  dimension "d344" = 10
  dimension "d345" = 10
  dimension "d346" = 10
  constraint concentric A41 A62
  constraint concentric A40 A63
  constraint concentric A39 A64
  constraint concentric A38 A65
  constraint concentric A37 A66
  constraint concentric A36 A67
  constraint concentric A21 A68
  constraint concentric A42 A69
  constraint concentric A25 A70
  constraint concentric A16 A71
  constraint concentric A10 A72
  constraint concentric A29 A73
  constraint concentric A22 A74
  constraint concentric A48 A75
  constraint concentric A26 A76
  constraint concentric A15 A77
  constraint concentric A35 A78
  constraint concentric A34 A79
  constraint concentric A33 A80
  constraint concentric A32 A81
  constraint concentric A31 A82
  constraint concentric A30 A83
  constraint concentric A35 A84
  constraint concentric A34 A85
  constraint concentric A80 A86
  constraint concentric A32 A87
  constraint concentric A82 A88
  constraint concentric A83 A89
  constraint concentric A72 A90
  constraint concentric A71 A91
  constraint concentric A70 A92
  constraint concentric A42 A93
  constraint concentric A68 A94
  constraint concentric A36 A95
  constraint concentric A66 A96
  constraint concentric A38 A97
  constraint concentric A39 A98
  constraint concentric A63 A99
  constraint concentric A41 A100
  constraint concentric A73 A101
  constraint concentric A74 A102
  constraint concentric A75 A103
  constraint concentric A26 A104
  constraint concentric A15 A105
  measures "d301" diameter of A62
  measures "d302" diameter of A63
  measures "d303" diameter of A64
  measures "d304" diameter of A65
  measures "d305" diameter of A66
  measures "d306" diameter of A67
  measures "d307" diameter of A68
  measures "d308" diameter of A69
  measures "d309" diameter of A70
  measures "d310" diameter of A71
  measures "d311" diameter of A72
  measures "d312" diameter of A73
  measures "d313" diameter of A74
  measures "d314" diameter of A75
  measures "d315" diameter of A76
  measures "d316" diameter of A77
  measures "d317" diameter of A78
  measures "d318" diameter of A79
  measures "d319" diameter of A80
  measures "d320" diameter of A81
  measures "d321" diameter of A82
  measures "d322" diameter of A83
  measures "d325" diameter of A84
  measures "d326" diameter of A85
  measures "d327" diameter of A86
  measures "d328" diameter of A87
  measures "d329" diameter of A88
  measures "d330" diameter of A89
  measures "d331" diameter of A90
  measures "d332" diameter of A91
  measures "d333" diameter of A92
  measures "d334" diameter of A93
  measures "d335" diameter of A94
  measures "d336" diameter of A95
  measures "d337" diameter of A96
  measures "d338" diameter of A97
  measures "d339" diameter of A98
  measures "d340" diameter of A99
  measures "d341" diameter of A100
  measures "d342" diameter of A101
  measures "d343" diameter of A102
  measures "d344" diameter of A103
  measures "d345" diameter of A104
  measures "d346" diameter of A105
extrude "Extrude2'''" cut sketch "Sketch2 (4)" against normal up to surface (10 mm away) contours A62 | A63 | A64 | A65 | A66 | A67 | A68 | A69 | A70 | A71 | A72 | A73 | A74 | A75 | A76 | A77 | A78 | A79 | A80 | A81 | A82 | A83 bodies 1
extrude "Extrude3'''" cut sketch "Sketch2 (4)" against normal blind 7 contours A84 | A85 | A86 | A87 | A88 | A89 | A90 | A91 | A92 | A93 | A94 | A95 | A96 | A97 | A98 | A99 | A100 | A101 | A102 | A103 | A104 | A105 bodies 1
extrude "Extrude4'" cut sketch "Sketch3 (2)" against normal blind 7 contours A16 | A17 bodies 2 in component "Back"
extrude "Extrude5'" cut 1 faces at (22.8333, 80.8833, 160) along direction (0, 0, -1) blind 101 on bodies 2 bodies 2 in component "Back"
extrude "Extrude8" cut 1 faces at (-61.8333, 70.8833, 160) along direction (0, 0, -1) blind 101 on bodies 3 bodies 3 in component "Side"
copy_body "Body->Comp1" bodies 1 removing the originals makes body 5 in component "Side v2"
component "Back" placed x (1, 0, 0) y (0, 1, 0) z (0, 0, 1) at (0, 0, 0)
component "Side" placed x (1, 0, 0) y (0, 1, 0) z (0, 0, 1) at (0, 0, 0)
component "Plate" placed x (1, 0, 0) y (0, 1, 0) z (0, 0, 1) at (0, 0, 0)
component "Side v2" placed x (1, 0, 0) y (0, 1, 0) z (0, 0, 1) at (0, 0, 0)
